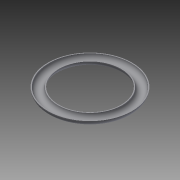
# Autodesk Inventor part: ring
Saved by Autodesk Inventor 2015 (Build 190159000, 159)
## iProperties
Created: 2016-03-12
Part Number: ring
Material: Generic
Document SubType Name: Modeling
Designer: Administrator
Density: 1 g/cm^3
Appearance: Default
Author: Administrator
Autodesk Inventor part; units mm, degrees
ref_plane "YZ Plane" through (0, 0, 0) normal (1, 0, 0) x (0, 1, 0)
ref_plane "XZ Plane" through (0, 0, 0) normal (0, 1, 0) x (-1, 0, 0)
ref_plane "XY Plane" through (0, 0, 0) normal (0, 0, 1) x (1, 0, 0)
sketch "Sketch3" plane through (0, 0, 0) normal (0, 0, 1) x (1, 0, 0)
  line L0 (0, 0) -> (-254, 0)
  circle A0 centre (-254, 0) radius 38.1
  circle A1 centre (-254, 0) radius 31.75
  line L1 (0, -53.34) -> (0, 53.34) projected
  dimension "centerRing" = 254
  dimension "outerDiam" = 76.2
  dimension "innerDiam" = 63.5
  constraints: 2 centre point, 2 coincident, 2 end point, 1 horizontal
  measures "centerRing" distance of L0.start L0.end
  measures "outerDiam" diameter of A0
  measures "innerDiam" diameter of A1
revolve "Revolution2" add sketch "Sketch3" angle 360 about axis through (0, -10, 0) along (0, 1, 0)
sketch "Sketch5" plane through (0, 0, 0) normal (0, 1, 0) x (-1, 0, 0)
  circle A0 centre (0, 0) radius 304.8
  dimension "removeDiam" = 609.6
  constraints: 1 centre point, 1 coincident
  measures "removeDiam" diameter of A0
extrude "Extrusion2" cut sketch "Sketch5" along normal through all
body "Solid2"
